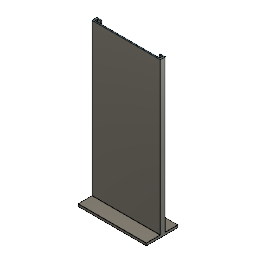
scannerstand v1 (Autodesk Fusion 360 design; units mm, degrees)
Autodesk Fusion 360 part; units mm, degrees
sketch "Sketch1" plane through (0, 0, 0) normal (0, 1, 0) x (1, 0, 0)
  line L0 (0, -10) -> (54, -10)
  line L1 (54, -10) -> (54, -14)
  line L2 (54, -14) -> (0, -14)
  line L3 (0, -14) -> (0, -10)
  line L4 (0, -10) -> (1.5, -10)
  line L5 (1.5, -11) -> (1.5, -12.5)
  line L6 (1.5, -14) -> (0, -14)
  line L7 (0, -14) -> (0, -10)
  line L8 (54, -10) -> (52.5, -10)
  line L9 (52.5, -11) -> (52.5, -12.5)
  line L10 (52.5, -14) -> (54, -14)
  line L11 (54, -14) -> (54, -10)
  line L12 (1.5, -14) -> (52.5, -14)
  line L13 (52.5, -12.5) -> (1.5, -12.5)
  line L14 (1.5, -10) -> (4, -10)
  line L15 (4, -10) -> (4, -11)
  line L16 (4, -11) -> (1.5, -11)
  line L17 (52.5, -10) -> (50, -10)
  line L18 (50, -10) -> (50, -11)
  line L19 (50, -11) -> (52.5, -11)
  dimension "d1" = 54
  dimension "d2" = 4
  dimension "d3" = 1.5
  dimension "d4" = 1.5
  dimension "d5" = 51
  dimension "d6" = 1.5
  constraint horizontal L0
  constraint vertical L1
  constraint horizontal L2
  constraint vertical L3
  constraint horizontal L4
  constraint vertical L5
  constraint horizontal L6
  constraint vertical L7
  constraint horizontal L8
  constraint vertical L9
  constraint horizontal L10
  constraint vertical L11
  constraint horizontal L12
  constraint horizontal L13
  constraint horizontal L14
  constraint vertical L15
  constraint horizontal L16
  constraint horizontal L17
  constraint vertical L18
  constraint horizontal L19
  measures "d1" distance of L0.start L0.end
  measures "d2" distance of L0.start L2.end
  measures "d3" distance of L0.start L4.end
  measures "d4" distance of L0.end L8.end
  measures "d5" distance of L6.start L10.start
  measures "d6" distance of L6.start L5.end
extrude "Extrude1" add sketch "Sketch1" along normal blind 120 contours L0 L1 L2 L3 L4 L5 L6 L7 L8 L9 L10 L11 L12 L13 L14 L15 L16 L17 L18 L19
sketch "Sketch2" plane through (0, 0, 0) normal (0, -1, 0) x (1, 0, 0)
  line L0 (54, 14) -> (0, 14)
  line L1 (0, 14) -> (0, 10)
  line L2 (0, 10) -> (4, 10)
  line L3 (4, 10) -> (4, 11)
  line L4 (4, 11) -> (1.5, 11)
  line L5 (1.5, 11) -> (1.5, 12.5)
  line L6 (1.5, 12.5) -> (52.5, 12.5)
  line L7 (52.5, 12.5) -> (52.5, 11)
  line L8 (52.5, 11) -> (50, 11)
  line L9 (50, 11) -> (50, 10)
  line L10 (50, 10) -> (54, 10)
  line L11 (54, 10) -> (54, 14)
  line L12 (0, 0) -> (54, 0)
  line L13 (54, 0) -> (54, 25)
  line L14 (54, 25) -> (0, 25)
  line L15 (0, 25) -> (0, 0)
  constraint horizontal L12
  constraint vertical L13
  constraint horizontal L14
  constraint vertical L15
  constraint coincident L12.start L15.end
extrude "Extrude2" add sketch "Sketch2" along normal blind 2
sketch "Sketch3" plane through (0, 120, 0) normal (0, 1, 0) x (-1, 0, 0)
  line L0 (0, 14) -> (-54, 14)
  line L1 (-54, 14) -> (-54, 10)
  line L2 (-54, 10) -> (-50, 10)
  line L3 (-50, 10) -> (-50, 11)
  line L4 (-50, 11) -> (-52.5, 11)
  line L5 (-52.5, 11) -> (-52.5, 12.5)
  line L6 (-52.5, 12.5) -> (-1.5, 12.5)
  line L7 (-1.5, 12.5) -> (-1.5, 11)
  line L8 (-1.5, 11) -> (-4, 11)
  line L9 (-4, 11) -> (-4, 10)
  line L10 (-4, 10) -> (0, 10)
  line L11 (0, 10) -> (0, 14)
  line L12 (-1.5, 12.5) -> (-52.5, 12.5)
  line L13 (-52.5, 12.5) -> (-52.5, 13)
  line L14 (-52.5, 13) -> (-1.5, 13)
  line L15 (-1.5, 13) -> (-1.5, 12.5)
  dimension "d11" = 0.5
  constraint horizontal L12
  constraint vertical L13
  constraint horizontal L14
  constraint vertical L15
  constraint coincident L6.end L7.start
  measures "d11" distance of L6.end L14.end
extrude "Extrude3" cut sketch "Sketch3" against normal blind 120 contours L6 L12 L13 L14 L15
sketch "Sketch4" plane through (0, 120, 0) normal (0, 1, 0) x (-1, 0, 0)
  line L0 (-1.5, 13) -> (-1.5, 11)
  line L1 (-1.5, 11) -> (-4, 11)
  line L2 (-4, 11) -> (-4, 10)
  line L3 (-4, 10) -> (0, 10)
  line L4 (0, 10) -> (0, 14)
  line L5 (0, 14) -> (-54, 14)
  line L6 (-54, 14) -> (-54, 10)
  line L7 (-54, 10) -> (-50, 10)
  line L8 (-50, 10) -> (-50, 11)
  line L9 (-50, 11) -> (-52.5, 11)
  line L10 (-52.5, 11) -> (-52.5, 13)
  line L11 (-52.5, 13) -> (-1.5, 13)
